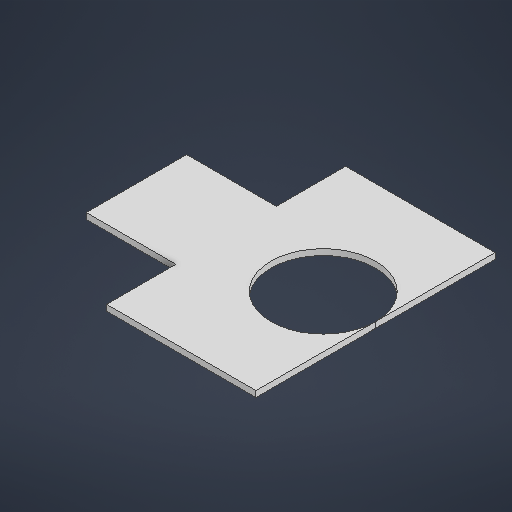
# Autodesk Inventor part: Base
Saved by Autodesk Inventor 2026.1 (Build 301233000, 233)
## iProperties
Created: 2026-07-03
Part Number: Base
Material: Generic
Document SubType Name: Modeling
Designer: Kasi Pusuluri
Density: 1 g/cm^3
Appearance: Default
Author: Kasi Pusuluri
Autodesk Inventor part; units mm, degrees
ref_plane "YZ Plane" through (0, 0, 0) normal (1, 0, 0) x (0, 1, 0)
ref_plane "XZ Plane" through (0, 0, 0) normal (0, 1, 0) x (-1, 0, 0)
ref_plane "XY Plane" through (0, 0, 0) normal (0, 0, 1) x (1, 0, 0)
sketch "Sketch1" plane through (0, 0, 0) normal (0, 1, 0) x (-1, 0, 0)
  line L0 (0, 0) -> (0, -25.4)
  line L1 (0, -25.4) -> (31.75, -25.4)
  line L2 (31.75, -25.4) -> (31.75, -10.668)
  line L3 (31.75, -10.668) -> (50.8, -10.668)
  line L4 (50.8, -10.668) -> (50.8, 10.668)
  line L5 (50.8, 10.668) -> (31.75, 10.668)
  line L6 (31.75, 10.668) -> (31.75, 25.4)
  line L7 (31.75, 25.4) -> (0, 25.4)
  line L8 (0, 25.4) -> (0, 0)
  line L9 (0, 0) -> (11.1125, 0)
  circle A0 centre (11.1125, 0) radius 11.1125
  dimension "d0" = 25.4
  dimension "d1" = 31.75
  dimension "d2" = 14.732
  dimension "d3" = 19.05
  dimension "d4" = 21.336
  dimension "d5" = 19.05
  dimension "d6" = 14.732
  dimension "d8" = 11.1125
  constraints: 20 end point, 4 horizontal, 3 vertical, 1 coincident, 1 collinear, 1 horizontal alignment, 1 perpendicular, 2 other
  measures "d0" distance of L0.start L0.end
  measures "d1" distance of L0.end L1.end
  measures "d2" distance of L1.end L2.end
  measures "d3" distance of L2.end L3.end
  measures "d4" distance of L3.end L4.end
  measures "d5" distance of L4.end L5.end
  measures "d6" distance of L5.end L6.end
  measures "d8" distance of L0.start L9.end
extrude "Extrusion1" add sketch "Sketch1" along normal blind 1.27
equation "\"d5\" = d3"
equation "\"d6\" = d2"
body "Solid1"
